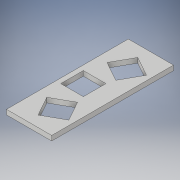
# Autodesk Inventor part: k2_t_top
Saved by Autodesk Inventor 2017 (Build 210142000, 142)
## iProperties
Created: 2017-02-08
Part Number: k2_t_top
Material: Generic
Document SubType Name: Modeling
Designer: herman
Density: 1 g/cm^3
Appearance: Default
Author: herman
Autodesk Inventor part; units mm, degrees
ref_plane "YZ Plane" through (0, 0, 0) normal (1, 0, 0) x (0, 1, 0)
ref_plane "XZ Plane" through (0, 0, 0) normal (0, 1, 0) x (-1, 0, 0)
ref_plane "XY Plane" through (0, 0, 0) normal (0, 0, 1) x (1, 0, 0)
sketch "Sketch2" plane through (0, 0, 0) normal (0, 1, 0) x (-1, 0, 0)
  line L0 (19.2111, 42.6505) -> (-8.7889, 42.6505)
  line L1 (-8.7889, 42.6505) -> (-8.7889, -32.8495)
  line L2 (-8.7889, -32.8495) -> (19.2111, -32.8495)
  line L3 (19.2111, -32.8495) -> (19.2111, 42.6505)
  dimension "d11" = 75.5
  dimension "d41" = 28
  constraints: 8 end point, 2 parallel, 1 horizontal, 1 perpendicular
  measures "d11" distance of L2.end L0.start
  measures "d41" distance of L1.end L2.end
extrude "Extrusion3" add sketch "Sketch2" along normal blind 3
sketch "Sketch6" plane through (0, 3, 0) normal (0, 1, 0) x (1, 0, 0)
  line L0 (-16.2111, -12.0368) -> (-2.2111, -12.0368)
  line L1 (-2.2111, -12.0368) -> (-2.2111, 1.9632)
  line L2 (-2.2111, 1.9632) -> (-16.2111, 1.9632)
  line L3 (-16.2111, 1.9632) -> (-16.2111, -12.0368)
  line L4 (-6.3559, -35.9231) -> (5.8695, -29.1012)
  line L5 (5.8695, -29.1012) -> (-0.9523, -16.8758)
  line L6 (-0.9523, -16.8758) -> (-13.1778, -23.6976)
  line L7 (-13.1778, -23.6976) -> (-6.3559, -35.9231)
  line L8 (-0.9523, 6.8022) -> (5.8695, 19.0276)
  line L9 (5.8695, 19.0276) -> (-6.3559, 25.8495)
  line L10 (-6.3559, 25.8495) -> (-13.1778, 13.6241)
  line L11 (-13.1778, 13.6241) -> (-0.9523, 6.8022)
  circle A0 centre (34.6298, -5.0368) radius 37.5 construction
  line L12 (-19.2111, 32.8495) -> (-19.2111, -42.6505) projected
  line L13 (8.7889, 32.8495) -> (-19.2111, 32.8495) projected
  point P0 (0, 0)
  dimension "d30" = 75
  dimension "d31" = 14
  dimension "d32" = 14
  dimension "d33" = 14
  dimension "d34" = 14
  dimension "d35" = 14
  dimension "d36" = 14
  dimension "d37" = 5
  dimension "d38" = 5
  dimension "d39" = 3
  dimension "d40" = 7
  constraints: 24 end point, 7 perpendicular, 6 point on circle, 2 parallel, 1 centre point, 1 horizontal
  measures "d30" diameter of A0
  measures "d31" distance of L0.start L0.end
  measures "d32" distance of L2.end L0.start
  measures "d33" distance of L5.end L6.end
  measures "d34" distance of L6.end L4.start
  measures "d35" distance of L9.end L10.end
  measures "d36" distance of L10.end L8.start
  measures "d37" distance of L0.end L5.end
  measures "d38" distance of L8.start L1.end
  measures "d39" distance between parallel lines of L12 L3
  measures "d40" distance from line of L13 L9.end
extrude "Extrusion4" cut sketch "Sketch6" against normal through all
body "Solid3"
